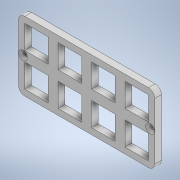
# Autodesk Inventor part: Plate
Saved by Autodesk Inventor 2020 (Build 240168000, 168)
## iProperties
Created: 2021-01-02
Part Number: Plate
Material: Generic
Document SubType Name: Modeling
Designer: user
Density: 1 g/cm^3
Appearance: Default
Author: user
Autodesk Inventor part; units mm, degrees
ref_plane "YZ Plane" through (0, 0, 0) normal (1, 0, 0) x (0, 1, 0)
ref_plane "XZ Plane" through (0, 0, 0) normal (0, 1, 0) x (-1, 0, 0)
ref_plane "XY Plane" through (0, 0, 0) normal (0, 0, 1) x (1, 0, 0)
sketch "Sketch2" plane through (0, 0, 0) normal (0, 0, 1) x (1, 0, 0)
  line L0 (0, 0) -> (14.1, 0)
  line L1 (14.1, 0) -> (14.1, 14.1)
  line L2 (14.1, 14.1) -> (0, 14.1)
  line L3 (0, 14.1) -> (0, 0)
  line L4 (20, 0) -> (34.1, 0)
  line L5 (34.1, 0) -> (34.1, 14.1)
  line L6 (34.1, 14.1) -> (20, 14.1)
  line L7 (20, 14.1) -> (20, 0)
  line L8 (40, 0) -> (54.1, 0)
  line L9 (54.1, 0) -> (54.1, 14.1)
  line L10 (54.1, 14.1) -> (40, 14.1)
  line L11 (40, 14.1) -> (40, 0)
  line L12 (60, 0) -> (74.1, 0)
  line L13 (74.1, 0) -> (74.1, 14.1)
  line L14 (74.1, 14.1) -> (60, 14.1)
  line L15 (60, 14.1) -> (60, 0)
  line L16 (0, -20) -> (14.1, -20)
  line L17 (14.1, -20) -> (14.1, -5.9)
  line L18 (14.1, -5.9) -> (0, -5.9)
  line L19 (0, -5.9) -> (0, -20)
  line L20 (20, -20) -> (34.1, -20)
  line L21 (34.1, -20) -> (34.1, -5.9)
  line L22 (34.1, -5.9) -> (20, -5.9)
  line L23 (20, -5.9) -> (20, -20)
  line L24 (40, -20) -> (54.1, -20)
  line L25 (54.1, -20) -> (54.1, -5.9)
  line L26 (54.1, -5.9) -> (40, -5.9)
  line L27 (40, -5.9) -> (40, -20)
  line L28 (60, -20) -> (74.1, -20)
  line L29 (74.1, -20) -> (74.1, -5.9)
  line L30 (74.1, -5.9) -> (60, -5.9)
  line L31 (60, -5.9) -> (60, -20)
  line L32 (0.05, 18.05) -> (74.05, 18.05)
  line L33 (78.05, 14.05) -> (78.05, -19.95)
  line L34 (74.05, -23.95) -> (0.05, -23.95)
  line L35 (-3.95, -19.95) -> (-3.95, 14.05)
  arc A0 (0.05, 18.05) -> (-3.95, 14.05) centre (0.05, 14.05) ccw
  arc A1 (-3.95, -19.95) -> (0.05, -23.95) centre (0.05, -19.95) ccw
  arc A2 (74.05, -23.95) -> (78.05, -19.95) centre (74.05, -19.95) ccw
  arc A3 (78.05, 14.05) -> (74.05, 18.05) centre (74.05, 14.05) ccw
  circle A4 centre (-0.95, -2.95) radius 1.15
  circle A5 centre (75.05, -2.95) radius 1.15
  point P0 (-3.95, 18.05)
  point P1 (78.05, -23.95)
  point P2 (78.05, 18.05)
  point P3 (-3.95, -23.95)
  dimension "d0" = 14.1
  dimension "d1" = 14.1
  dimension "d6" = 20
  dimension "d9" = 20
  dimension "d18" = 4
  dimension "d19" = 2.3
  dimension "d20" = 3
  dimension "d22" = 21
  dimension "d23" = 42
  dimension "d24" = 82
  dimension "d25" = 3
  dimension "d26" = 21
  dimension "d27" = 23.95
  dimension "d28" = 38.05
  constraints: 72 end point, 8 point on circle, 8 point on line, 8 tangent, 6 centre point, 4 parallel, 3 equal radius, 3 horizontal, 2 collinear, 2 perpendicular, 1 vertical, 54 other
  measures "d0" distance of L2.end L1.end
  measures "d1" distance of L1.end L0.end
  measures "d6" distance of L1.end L5.end
  measures "d9" distance of L1.end L17.end
  measures "d18" radius of A0
  measures "d19" diameter of A4
  measures "d20" distance from line of L35 A4.centre
  measures "d22" distance from line of L34 A4.centre
  measures "d23" distance between parallel lines of L34 L32
  measures "d24" distance between parallel lines of L35 L33
  measures "d25" distance from line of A5.centre L33
  measures "d26" distance from line of L34 A5.centre
  measures "d27" distance between parallel lines of L34 L4
  measures "d28" distance between parallel lines of L35 L5
extrude "Extrusion1" add sketch "Sketch2" along normal blind 4
chamfer "Chamfer1" distance 1.5 angle 45 2 edges at (-2.1, -2.95, 4) (73.9, -2.95, 4)
sketch "Sketch3" plane through (0, 0, 4) normal (0, 0, 1) x (1, 0, 0)
  line L0 (0.05, 18.05) -> (74.05, 18.05)
  line L1 (78.05, 14.05) -> (78.05, -19.95)
  line L2 (74.05, -23.95) -> (0.05, -23.95)
  line L3 (-3.95, -19.95) -> (-3.95, 14.05)
  arc A0 (0.05, 18.05) -> (-3.95, 14.05) centre (0.05, 14.05) ccw
  arc A1 (-3.95, -19.95) -> (0.05, -23.95) centre (0.05, -19.95) ccw
  arc A2 (74.05, -23.95) -> (78.05, -19.95) centre (74.05, -19.95) ccw
  arc A3 (78.05, 14.05) -> (74.05, 18.05) centre (74.05, 14.05) ccw
  line L4 (74.05, 17.75) -> (0.05, 17.75)
  arc A4 (0.05, 17.75) -> (-3.65, 14.05) centre (0.05, 14.05) ccw
  line L5 (-3.65, 14.05) -> (-3.65, -19.95)
  arc A5 (-3.65, -19.95) -> (0.05, -23.65) centre (0.05, -19.95) ccw
  line L6 (0.05, -23.65) -> (74.05, -23.65)
  arc A6 (74.05, -23.65) -> (77.75, -19.95) centre (74.05, -19.95) ccw
  line L7 (77.75, -19.95) -> (77.75, 14.05)
  arc A7 (77.75, 14.05) -> (74.05, 17.75) centre (74.05, 14.05) ccw
  point P0 (0, 0)
  dimension "d32" = 4
  dimension "d33" = 0.3
  constraints: 16 end point, 16 point on circle, 8 centre point, 8 tangent, 4 parallel, 3 equal radius, 2 perpendicular, 1 horizontal, 7 other
  measures "d32" radius of A0
  measures "d33" distance between parallel lines of L0 L4
extrude "Extrusion2" cut sketch "Sketch3" against normal blind 10
body "Solid1"
